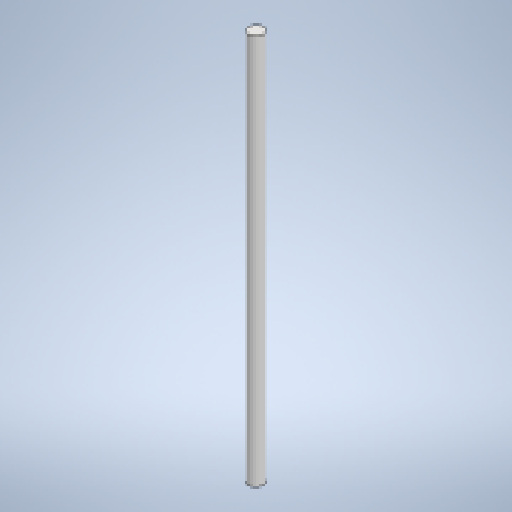
# Autodesk Inventor part: TRM 028 main shaft
Saved by Autodesk Inventor 2025 (Build 290162010, 162A)
## iProperties
Created: 2024-09-08
Part Number: TRM 028 main shaft
Material: Generic
Document SubType Name: Modeling
Designer: admin
Density: 1 g/cm^3
Appearance: Default
Author: admin
Autodesk Inventor part; units mm, degrees
ref_plane "YZ Plane" through (0, 0, 0) normal (1, 0, 0) x (0, 1, 0)
ref_plane "XZ Plane" through (0, 0, 0) normal (0, 1, 0) x (-1, 0, 0)
ref_plane "XY Plane" through (0, 0, 0) normal (0, 0, 1) x (1, 0, 0)
sketch "Sketch1" plane through (0, 0, 0) normal (0, 1, 0) x (-1, 0, 0)
  line L0 (0, 0) -> (0, 300)
  line L1 (0, 300) -> (-12.5, 300)
  line L2 (-12.5, 300) -> (-12.5, 0)
  line L3 (-12.5, 0) -> (-12.5, -400)
  line L4 (-12.5, -400) -> (0, -400)
  line L5 (0, -400) -> (0, 0)
  dimension "d0" = 25
  dimension "d1" = 300
  dimension "d2" = 400
  constraints: 12 end point, 3 perpendicular, 2 point on line, 1 collinear, 1 horizontal alignment, 1 vertical
  measures "d0" diameter of L2 L0
  measures "d1" distance of L1.end L2.end
  measures "d2" distance of L2.end L3.end
revolve "Revolution1" add sketch "Sketch1" angle 360 about axis through (0, 0, 0) along (0, 0, 1)
body "Solid1"
